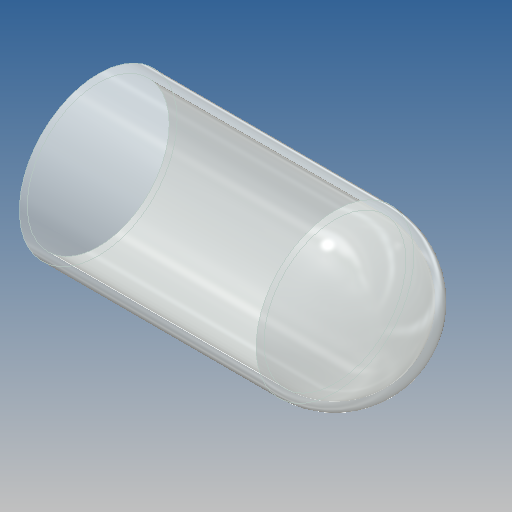
# Autodesk Inventor part: Verdrängerkolben
Saved by Autodesk Inventor 2018 (Build 220112000, 112)
## iProperties
Created: 2018-10-02
Part Number: Verdrängerkolben
Material: Glas
Document SubType Name: Modeling
Designer: M.Knabel
Density: 2.18 g/cm^3
Appearance: Klar
Mass: 8.88377 g
Surface Area: 68.8084 cm^2
Volume: 4.07512 cm^3
Author: M.Knabel
Autodesk Inventor part; units mm, degrees
ref_plane "YZ Plane" through (0, 0, 0) normal (1, 0, 0) x (0, 1, 0)
ref_plane "XZ Plane" through (0, 0, 0) normal (0, 1, 0) x (-1, 0, 0)
ref_plane "XY Plane" through (0, 0, 0) normal (0, 0, 1) x (1, 0, 0)
sketch "Skizze1" plane through (0, 0, 0) normal (0, 0, 1) x (1, 0, 0)
  line L0 (0, -2.8971) -> (0, 17.3823) projected
  line L1 (-10.0971, 0) -> (60.5823, 0) projected
  line L2 (0, 12) -> (36, 12)
  arc A0 (48, 0) -> (36, 12) centre (36, 0) ccw
  line L3 (0, 12) -> (0, 10.8)
  line L4 (0, 10.8) -> (36, 10.8)
  arc A1 (46.8, 0) -> (36, 10.8) centre (36, 0) ccw
  line L5 (46.8, 0) -> (48, 0)
  point P0 (0, 0)
  dimension "d0" = 24
  dimension "d1" = 21.6
  dimension "d2" = 12
  dimension "d4" = 1.2
  dimension "d5" = 48
  dimension "d6" = 46.8
  constraints: 8 end point, 4 point on circle, 4 point on line, 2 centre point, 2 horizontal, 1 concentric, 1 tangent
  measures "d0" diameter of L2 L1
  measures "d1" diameter of L4 L1
  measures "d2" radius of A0
  measures "d4" distance between parallel lines of L4 L2
  measures "d5" distance from line of L5.end L0
  measures "d6" distance from line of L0 L5.start
revolve "Umdrehung1" add sketch "Skizze1" angle 360 about axis through (-10, 0, 0) along (1, 0, 0) contours L0 L2 A0 L1 A1 L4
